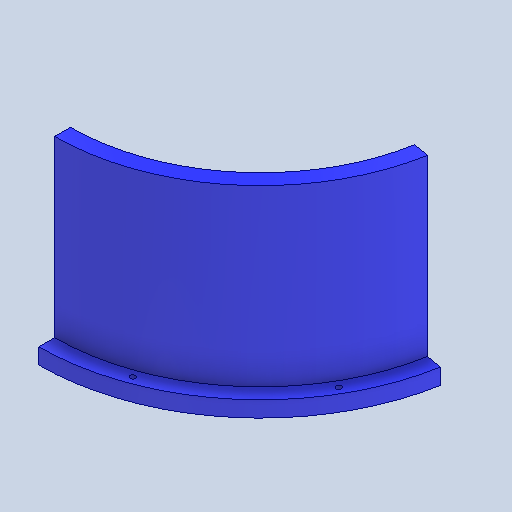
# Autodesk Inventor part: belt_liner_v1_3DP_C_B_U
Saved by Autodesk Inventor 2025.1 (Build 291241000, 241)
## iProperties
Created: 2024-12-14
Part Number: belt_liner_v1_3DP_C_B_U
Material: ABS プラスチック
Document SubType Name: Modeling
Designer: haruy
Density: 1.06 g/cm^3
Appearance: 青 - 壁塗料 - 光沢
Author: haruy
Autodesk Inventor part; units mm, degrees
ref_plane "YZ Plane" through (0, 0, 0) normal (1, 0, 0) x (0, 1, 0)
ref_plane "XZ Plane" through (0, 0, 0) normal (0, 1, 0) x (-1, 0, 0)
ref_plane "XY Plane" through (0, 0, 0) normal (0, 0, 1) x (1, 0, 0)
sketch "スケッチ1" plane through (0, 0, 0) normal (1, 0, 0) x (0, 1, 0)
  circle A0 centre (0, 0) radius 120
  circle A1 centre (0, 0) radius 130
  line L0 (0, 0) -> (84.8528, 84.8528)
  line L1 (0, 0) -> (0, 120)
  line L2 (84.8528, 84.8528) -> (91.9239, 91.9239)
  line L3 (-130, 237.6299) -> (-130, -340.0687)
  line L4 (58.9191, 140) -> (-130, 140)
  line L5 (0, 0) -> (-130, 0)
  line L6 (0, 120) -> (0, 130)
  line L7 (-120, 140) -> (-120, 130)
  line L8 (-120, 130) -> (0, 130)
  line L9 (-120, 0) -> (-120, 140)
  line L10 (-110, 140) -> (-110, 130)
  point P0 (-120, 0)
  dimension "d0" = 240
  dimension "d1" = 10
  dimension "d2" = 45
  dimension "d3" = 140
  dimension "d4" = 0
  dimension "d5" = 10
  dimension "d6" = 10
  dimension "d8" = 10
  constraints: 22 end point, 6 point on circle, 6 point on line, 3 vertical, 2 centre point, 1 coincident, 1 collinear, 1 parallel, 1 perpendicular, 1 tangent
  measures "d0" diameter of A0
  measures "d1" radial gap between concentric circles of A0 A1
  measures "d3" distance between parallel lines of L4 L5
  measures "d4" distance from line of L1 L6.end
  measures "d5" distance of L7.start L7.end
  measures "d6" distance between parallel lines of L7 L3
  measures "d8" distance between parallel lines of L9 L10
revolve "回転1" add sketch "スケッチ1" angle 80 about axis through (0, 0, 0) along (0, 1, 0) contours L9 A1 L6 A0 | L9 L8 A1 | L7 L4 L10 L8
sketch "スケッチ2" plane through (0, -110, 140) normal (0, 1, 0) x (1, 0, 0)
  line L0 (137.8731, 115.6893) -> (0, 140) projected
  line L1 (0, 0) -> (0, 140) projected
  circle A0 centre (0, 140) radius 140
  circle A1 centre (0, 140) radius 135
  point P0 (46.1727, 13.1415)
  point P1 (116.9134, 72.5)
  dimension "d9" = 5
  dimension "d10" = 20
  dimension "d11" = 20
  constraints: 2 point on circle, 1 centre point, 1 coincident, 1 vertical alignment, 2 other
hole "穴1" at (46.1727, -110, 126.8585) at (116.9134, -110, 67.5) direction (0, -1, 0) diameter 3.4 end through all
sketch "スケッチ3" plane through (0, -120, 0) normal (0, -1, 0) x (1, 0, 0)
  line L0 (17, -30) -> (-17, -30)
  line L1 (-17, -30) -> (-17, 30)
  line L2 (-17, 30) -> (17, 30)
  line L3 (17, 30) -> (17, -30)
  circle A0 centre (14.5, 7.5) radius 4
  point P0 (0, 0)
  point P1 (17, 10.6225)
  point P2 (17, 4.3775)
  dimension "d19" = 34
  dimension "d20" = 60
  dimension "d21" = 30
  dimension "d22" = 17
  dimension "d25" = 8
  dimension "d26" = 2.5
  dimension "d27" = 22.5
  constraints: 8 end point, 2 parallel, 1 centre point, 1 horizontal, 1 perpendicular
  measures "d19" distance of L1.end L2.end
  measures "d20" distance of L0.end L1.end
  measures "d21" distance from line of L2 point (0, 0)
  measures "d22" distance from line of point (0, 0) L3
  measures "d25" diameter of A0
  measures "d26" distance from line of A0.centre L3
  measures "d27" distance from line of L2 A0.centre
extrude "押し出し1" cut sketch "スケッチ3" against normal blind 10
fillet "フィレット2" radius 2 5 edges at (17, -119.376, 2.9976) (17, -119.3545, 4.3775) (17, -119.1569, 10.6225) (17, -117.4696, 30) (0, -118.0948, 30)
